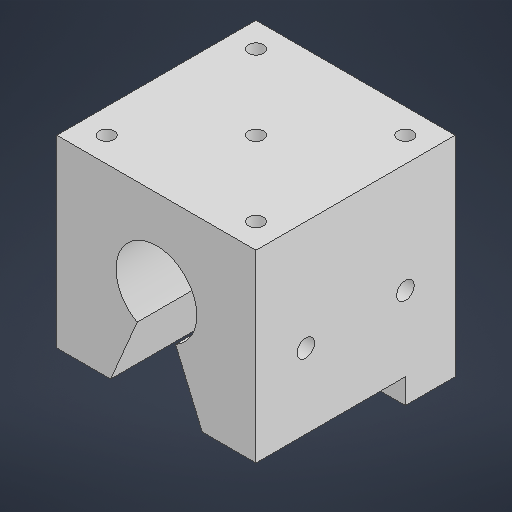
# Autodesk Inventor part: X Axis End
Saved by Autodesk Inventor 2025.1 (Build 291241000, 241)
## iProperties
Created: 2024-11-25
Part Number: X Axis End
Material: Generic
Document SubType Name: Modeling
Designer: jerem
Density: 1 g/cm^3
Appearance: Default
Author: jerem
## iProperties of the stored document X Axis End_3DPrint.ipt
Created: 2025-02-03
Part Number: X Axis End_3DPrint
Material: Generic
Document SubType Name: Modeling
Designer: jerem
Density: 1 g/cm^3
Appearance: Default
Author: jerem
Autodesk Inventor part; units mm, degrees
ref_plane "YZ Plane" through (0, 0, 0) normal (1, 0, 0) x (0, 1, 0)
ref_plane "XZ Plane" through (0, 0, 0) normal (0, 1, 0) x (-1, 0, 0)
ref_plane "XY Plane" through (0, 0, 0) normal (0, 0, 1) x (1, 0, 0)
sketch "Sketch1" plane through (0, 0, 0) normal (0, 0, 1) x (1, 0, 0)
  circle A0 centre (0, 24.7) radius 8.1
  line L0 (0, 24.7) -> (0, 0) construction
  line L1 (0, 0) -> (-20, 0) construction
  line L2 (-20, 5) -> (-9.2, 5)
  line L3 (-9.2, 5) -> (-3.85, 17.5735)
  line L4 (0, 0) -> (20, 0) construction
  line L5 (20, 0) -> (20, 5) construction
  line L6 (20, 5) -> (9.2, 5)
  line L7 (9.2, 5) -> (3.85, 17.5735)
  line L8 (0, 24.7) -> (0, 32.8) construction
  line L9 (-3.85, 17.5735) -> (3.85, 17.5735) construction
  line L10 (-20, 5) -> (-20, 42)
  line L11 (-20, 42) -> (20, 42)
  line L12 (20, 42) -> (20, 5)
  line L13 (-20, 5) -> (-20, 0)
  line L14 (-20, 0) -> (20, 0)
  line L15 (20, 0) -> (20, 5)
  line L16 (-9.2, 5) -> (9.2, 5)
  point P0 (0, 42)
  point P1 (-20, 5)
  dimension "d0" = 16.2
  dimension "d2" = 5
  dimension "d5" = 7.7
  dimension "d91" = 42
  dimension "d102" = 19.7
  dimension "d103" = 18.4
  dimension "d104" = 40
  constraints: 34 end point, 4 horizontal, 4 perpendicular, 4 vertical, 3 equal length, 3 point on circle, 2 coincident, 2 midpoint, 1 centre point, 1 parallel
  measures "d0" diameter of A0
  measures "d2" distance of L1.end L2.start
  measures "d5" distance of L9.start L7.end
  measures "d91" distance between parallel lines of L1 L11
  measures "d102" distance from line of L6 point (0, 24.7)
  measures "d103" distance of L3.start L6.end
  measures "d104" distance of L4.end L1.end
extrude "Extrusion1" add sketch "Sketch1" along normal blind 30 contours A0 L3 L2 L10 L11 L12 L6 L7
extrude "Extrusion2" add sketch "Sketch1" against normal blind 10
sketch "Sketch6" plane through (-20, 42, 30) normal (0, 1, 0) x (1, 0, 0)
  line L0 (0, 40) -> (0, 0) projected
  line L1 (40, 0) -> (0, 0) projected
  line L2 (0, 40) -> (40, 0) construction
  line L3 (40, 40) -> (0, 0) construction
  circle A0 centre (35, 5) radius 1.5
  circle A1 centre (5, 5) radius 1.5
  circle A2 centre (5, 35) radius 1.5
  circle A3 centre (35, 35) radius 1.5
  line L4 (35, 35) -> (35, 5) construction
  line L5 (5, 5) -> (35, 5) construction
  line L6 (5, 5) -> (5, 35) construction
  circle A4 centre (20, 20) radius 1.5
  line L7 (40, 40) -> (40, 0) projected
  line L8 (0, 40) -> (40, 40) projected
  point P0 (20, 30)
  dimension "d69" = 30
  dimension "d70" = 3
  dimension "d73" = 3
  constraints: 10 end point, 5 centre point, 4 point on line, 3 equal radius, 3 perpendicular, 2 midpoint, 1 coincident
  measures "d69" distance of L6.start L5.end
  measures "d70" diameter of A0
  measures "d73" diameter of A4
extrude "Extrusion8" cut sketch "Sketch6" against normal blind 5 contours A0 | A1 | A2 | A3
extrude "Extrusion9" cut sketch "Sketch6" against normal through all contours A4
sketch "Sketch8" plane through (20, 5, 30) normal (1, 0, 0) x (0, 0, -1)
  line L0 (0, 0) -> (0, 37) projected
  line L1 (30, 0) -> (0, 0) projected
  line L2 (20, 37) -> (20, 15) construction
  line L3 (20, 15) -> (10, 15) construction
  line L4 (20, 15) -> (30, 15) construction
  circle A0 centre (10, 15) radius 1.75
  circle A1 centre (30, 15) radius 1.75
  line L5 (40, 37) -> (0, 37) projected
  line L6 (30, -5) -> (30, 0) projected
  line L7 (30, -5) -> (40, -5) projected
  line L8 (40, 37) -> (40, -5) projected
  point P0 (30, -5)
  point P1 (35, -5)
  dimension "d97" = 3.5
  dimension "d98" = 3.5
  dimension "d105" = 20
  dimension "d106" = 20
  dimension "d107" = 20
  constraints: 6 end point, 2 centre point, 2 coincident, 1 collinear, 1 horizontal, 1 midpoint, 1 perpendicular, 1 vertical
  measures "d97" diameter of A0
  measures "d98" diameter of A1
  measures "d105" distance from line of point (35, -5) L4
  measures "d106" distance of L4.end L3.end
  measures "d107" distance between parallel lines of L0 L2
extrude "Extrusion12" cut sketch "Sketch8" against normal blind 5 contours A0 | A1
mirror "Mirror1" about plane through (0, 0, 0) normal (1, 0, 0) of "Extrusion12"
body "Solid1"
